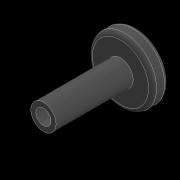
# Autodesk Inventor part: BottomStandoffs
Saved by Autodesk Inventor 2022 (Build 260153000, 153)
## iProperties
Created: 2023-01-19
Part Number: BottomStandoffs
Material: Custom TPU
Document SubType Name: Modeling
Designer: tandu
Density: 1.21 g/cm^3
Appearance: Generic
Author: tandu
Autodesk Inventor part; units mm, degrees
ref_plane "YZ Plane" through (0, 0, 0) normal (1, 0, 0) x (0, 1, 0)
ref_plane "XZ Plane" through (0, 0, 0) normal (0, 1, 0) x (-1, 0, 0)
ref_plane "XY Plane" through (0, 0, 0) normal (0, 0, 1) x (1, 0, 0)
sketch "Sketch1" plane through (0, 0, 0) normal (0, 0, 1) x (1, 0, 0)
  circle A0 centre (0, 0) radius 2.5
  circle A1 centre (0, 0) radius 1.5
  circle A2 centre (0, 0) radius 6.35
  dimension "d0" = 5
  dimension "d1" = 3
  dimension "d2" = 12.7
  constraints: 3 centre point, 3 coincident
  measures "d0" diameter of A0
  measures "d1" diameter of A1
  measures "d2" diameter of A2
extrude "Extrusion1" add sketch "Sketch1" along normal blind 15.24 contours A0
extrude "Extrusion2" add sketch "Sketch1" against normal blind 3.175 contours A0 | A2
fillet "Fillet1" radius 0.7937 2 edges at (-6.35, 0, 0) (-6.35, 0, -3.175)
body "Solid1"
